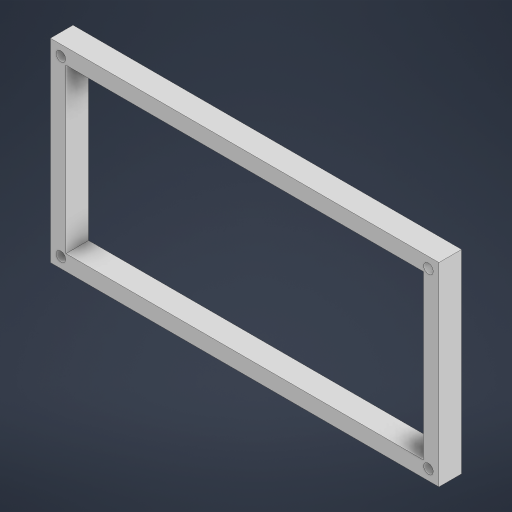
# Autodesk Inventor part: rack_C2x1
Saved by Autodesk Inventor 2024 (Build 280153000, 153)
## iProperties
Created: 2026-04-07
Part Number: rack_C2x1
Material: Generic
Document SubType Name: Modeling
Designer: schar
Density: 1 g/cm^3
Appearance: Default
Author: schar
Autodesk Inventor part; units mm, degrees
ref_plane "YZ Plane" through (0, 0, 0) normal (1, 0, 0) x (0, 1, 0)
ref_plane "XZ Plane" through (0, 0, 0) normal (0, 1, 0) x (-1, 0, 0)
ref_plane "XY Plane" through (0, 0, 0) normal (0, 0, 1) x (1, 0, 0)
sketch "Sketch1" plane through (0, 0, 0) normal (0, 0, 1) x (1, 0, 0)
  line L0 (-25.2, 25.2) -> (25.2, 25.2)
  line L1 (25.2, 25.2) -> (25.2, -25.2)
  line L2 (25.2, -25.2) -> (-25.2, -25.2)
  line L3 (-25.2, -25.2) -> (-25.2, 25.2)
  line L4 (-25.2, 25.2) -> (25.2, -25.2) construction
  line L5 (25.2, 25.2) -> (-25.2, -25.2) construction
  line L6 (-30, 30) -> (30, 30)
  line L7 (30, 30) -> (30, -30)
  line L8 (30, -30) -> (-30, -30)
  line L9 (-30, -30) -> (-30, 30)
  line L10 (-30, 30) -> (30, -30) construction
  line L11 (30, 30) -> (-30, -30) construction
  line L12 (-30, 30) -> (-26.768, 30)
  line L13 (-26.768, 30) -> (-26.768, 26.768)
  circle A0 centre (-26.768, 26.768) radius 1.5
  circle A1 centre (-26.768, -26.768) radius 1.5
  circle A2 centre (26.768, -26.768) radius 1.5
  circle A3 centre (26.768, 26.768) radius 1.5
  line L14 (85.2, 25.2) -> (34.8, 25.2)
  line L15 (34.8, 25.2) -> (34.8, -25.2)
  line L16 (34.8, -25.2) -> (85.2, -25.2)
  line L17 (85.2, -25.2) -> (85.2, 25.2)
  line L18 (85.2, 25.2) -> (34.8, -25.2) construction
  line L19 (34.8, 25.2) -> (85.2, -25.2) construction
  line L20 (90, 30) -> (30, 30)
  line L21 (30, -30) -> (90, -30)
  line L22 (90, -30) -> (90, 30)
  line L23 (90, 30) -> (30, -30) construction
  line L24 (30, 30) -> (90, -30) construction
  line L25 (90, 30) -> (86.768, 30)
  line L26 (86.768, 30) -> (86.768, 26.768)
  circle A4 centre (86.768, 26.768) radius 1.5
  circle A5 centre (86.768, -26.768) radius 1.5
  line L27 (25.2, 25.2) -> (34.8, 25.2)
  line L28 (25.2, -25.2) -> (34.8, -25.2)
  point P0 (0, 0)
  point P1 (60, 0)
  dimension "d0" = 50.4
  dimension "d1" = 50.4
  dimension "d2" = 60
  dimension "d3" = 60
  dimension "d4" = 3.232
  dimension "d5" = 3.232
  dimension "d6" = 3
  dimension "d9" = 360
  constraints: 58 end point, 11 symmetric about line, 6 centre point, 5 parallel, 5 point on line, 4 midpoint, 2 coincident, 2 horizontal, 2 perpendicular, 11 other
  measures "d0" distance of L1.end L2.end
  measures "d1" distance of L0.end L1.end
  measures "d2" distance of L7.end L8.end
  measures "d3" distance of L6.end L7.end
  measures "d4" distance of L6.start L12.end
  measures "d5" distance of L12.end L13.end
  measures "d6" diameter of A0
extrude "Extrusion1" add sketch "Sketch1" along normal blind 7 contours L3 L2 L28 L7 L8 L9 L6 L27 L0 | L7 L20 L22 L21 L28 L16 L17 L14 L27 | A2 | A3
body "Solid1"
